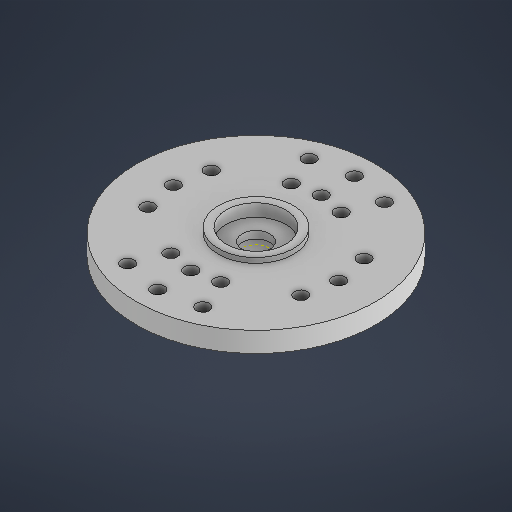
# Autodesk Inventor part: MMAE 232 CAD Assignment 2 Servo Horn 4-Nicholas Skiba
Saved by Autodesk Inventor 2026.1 (Build 301233000, 233)
## iProperties
Created: 2025-08-27
Part Number: MMAE 232 CAD Assignment 2 Servo Horn 4-Nicholas Skiba
Material: Generic
Document SubType Name: Modeling
Designer: Nick
Density: 1 g/cm^3
Appearance: Default
Author: Nick
Autodesk Inventor part; units mm, degrees
ref_plane "YZ Plane" through (0, 0, 0) normal (1, 0, 0) x (0, 1, 0)
ref_plane "XZ Plane" through (0, 0, 0) normal (0, 1, 0) x (-1, 0, 0)
ref_plane "XY Plane" through (0, 0, 0) normal (0, 0, 1) x (1, 0, 0)
sketch "Sketch1" plane through (0, 0, 0) normal (0, 1, 0) x (-1, 0, 0)
  circle A0 centre (0, 0) radius 11.915
  dimension "d0" = 23.83
  constraints: 1 centre point, 1 coincident
  measures "d0" diameter of A0
extrude "Extrusion1" add sketch "Sketch1" along normal blind 2
sketch "Sketch2" plane through (0, 2, 0) normal (0, 1, 0) x (1, 0, 0)
  circle A0 centre (0, 0) radius 3.73
  circle A1 centre (0, 0) radius 2.97
  circle A2 centre (0, 0) radius 1.37
  dimension "d3" = 7.46
  dimension "d4" = 5.94
  dimension "d5" = 2.74
  constraints: 3 centre point, 3 coincident
  measures "d3" diameter of A0
  measures "d4" diameter of A1
  measures "d5" diameter of A2
extrude "Extrusion2" add sketch "Sketch2" along normal blind 0.5 contours A0
extrude "Extrusion3" cut sketch "Sketch2" against normal blind 0.75 contours A1
extrude "Extrusion4" cut sketch "Sketch2" against normal through all contours A2
sketch "Sketch3" plane through (0, 0, 0) normal (0, -1, 0) x (1, 0, 0)
  circle A0 centre (0, 0) radius 4.44
  circle A1 centre (0, 0) radius 2.75
  dimension "d12" = 8.88
  dimension "d13" = 5.5
  constraints: 2 centre point, 2 coincident
  measures "d12" diameter of A0
  measures "d13" diameter of A1
extrude "Extrusion5" add sketch "Sketch3" along normal blind 2.5
extrude "Extrusion6" cut sketch "Sketch3" against normal blind 0.5 contours A1
sketch "Sketch4" plane through (0, 0, 0) normal (0, -1, 0) x (1, 0, 0)
  circle A0 centre (0, 0) radius 4.44 construction
  circle A1 centre (0, 0) radius 9.8 construction
  circle A2 centre (0, 0) radius 1.37 construction
  circle A3 centre (0, 0) radius 8.25 construction
  circle A4 centre (0, 0) radius 6.5 construction
  circle A5 centre (0, 0) radius 11.915 construction
  line L0 (0, 11.915) -> (0, -11.915) construction
  line L1 (-13.7871, 0) -> (13.3861, 0) construction
  circle A6 centre (0, 0) radius 3.73 construction
  line L2 (0, 0) -> (-5.9338, -14.3254) construction
  line L3 (0, 0) -> (5.2891, -12.7691) construction
  line L4 (0, 0) -> (12.9454, -5.3622) construction
  line L5 (0, 0) -> (13.6262, 5.6441) construction
  circle A7 centre (2.4874, -6.0052) radius 0.65
  circle A8 centre (3.7503, -9.054) radius 0.65
  circle A9 centre (-3.7503, -9.054) radius 0.65
  circle A10 centre (0, -9.8) radius 0.65
  circle A11 centre (0, -6.5) radius 0.65
  circle A12 centre (-2.4874, -6.0052) radius 0.65
  circle A13 centre (7.622, -3.1571) radius 0.65
  circle A14 centre (8.25, 0) radius 0.65
  circle A15 centre (7.622, 3.1571) radius 0.65
  circle A16 centre (2.4874, 6.0052) radius 0.65
  circle A17 centre (3.7503, 9.054) radius 0.65
  circle A18 centre (-3.7503, 9.054) radius 0.65
  circle A19 centre (0, 9.8) radius 0.65
  circle A20 centre (0, 6.5) radius 0.65
  circle A21 centre (-2.4874, 6.0052) radius 0.65
  circle A22 centre (-7.622, -3.1571) radius 0.65
  circle A23 centre (-8.25, 0) radius 0.65
  circle A24 centre (-7.622, 3.1571) radius 0.65
  dimension "d18" = 19.6
  dimension "d19" = 16.5
  dimension "d20" = 13
  dimension "d21" = 22.5
  dimension "d22" = 22.5
  dimension "d23" = 22.5
  dimension "d24" = 22.5
  dimension "d25" = 1.3
  dimension "d26" = 1.3
  dimension "d27" = 1.3
  dimension "d28" = 1.3
  dimension "d29" = 1.3
  dimension "d30" = 1.3
  dimension "d31" = 1.3
  dimension "d32" = 1.3
  dimension "d33" = 1.3
  constraints: 21 centre point, 12 end point, 11 point on circle, 9 point on line, 9 symmetric about line, 3 coincident, 1 perpendicular, 1 vertical, 9 other
  measures "d18" diameter of A1
  measures "d19" diameter of A3
  measures "d20" diameter of A4
  measures "d21" angle of L0 L3
  measures "d22" angle of L0 L2
  measures "d23" angle of L1 L4
  measures "d24" angle of L1 L5
  measures "d25" diameter of A7
  measures "d26" diameter of A8
  measures "d27" diameter of A9
  measures "d28" diameter of A10
  measures "d29" diameter of A11
  measures "d30" diameter of A12
  measures "d31" diameter of A13
  measures "d32" diameter of A14
  measures "d33" diameter of A15
sketch "Sketch5" plane through (0, 0, 0) normal (0, -1, 0) x (1, 0, 0)
  circle A0 centre (0, 0) radius 1.37 construction
  circle A1 centre (0, 0) radius 2.97 construction
extrude "Extrusion7" cut sketch "Sketch4" against normal through all
body "Solid1"
